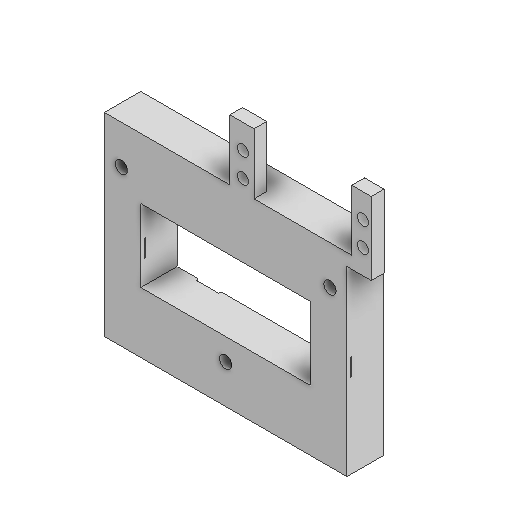
# Autodesk Inventor part: płytka_prowadzaca_rysik
Saved by Autodesk Inventor 2025.1 (Build 291241000, 241)
## iProperties
Created: 2025-04-08
Part Number: płytka_prowadzaca_rysik
Material: Ogólny
Document SubType Name: Modeling
Designer: Maciej
Density: 1 g/cm^3
Appearance: Domyślna
Author: Maciej
Autodesk Inventor part; units mm, degrees
ref_plane "YZ Plane" through (0, 0, 0) normal (1, 0, 0) x (0, 1, 0)
ref_plane "XZ Plane" through (0, 0, 0) normal (0, 1, 0) x (-1, 0, 0)
ref_plane "XY Plane" through (0, 0, 0) normal (0, 0, 1) x (1, 0, 0)
sketch "Szkic5" plane through (0, 0, 0) normal (0, 0, 1) x (1, 0, 0)
  line L0 (-50, -40) -> (50, -40)
  line L1 (50, -40) -> (50, 40)
  line L2 (50, 40) -> (-50, 40)
  line L3 (-50, 40) -> (-50, -40)
  line L4 (-50, -40) -> (50, 40) construction
  line L5 (50, -40) -> (-50, 40) construction
  line L6 (-35, -25) -> (35, -25)
  line L7 (35, -25) -> (35, 25)
  line L8 (35, 25) -> (-35, 25)
  line L9 (-35, 25) -> (-35, -25)
  line L10 (-35, -25) -> (35, 25) construction
  line L11 (35, -25) -> (-35, 25) construction
  point P0 (0, 0)
  dimension "d27" = 100
  dimension "d28" = 80
  dimension "d29" = 70
  dimension "d30" = 50
  constraints: 24 end point, 4 midpoint, 4 parallel, 2 horizontal, 2 perpendicular
  measures "d27" distance of L2.end L1.end
  measures "d28" distance of L1.end L0.end
  measures "d29" distance of L8.end L7.end
  measures "d30" distance of L7.end L6.end
extrude "Wyciągnięcie proste4" add sketch "Szkic5" against normal blind 13
sketch "Szkic6" plane through (0, 0, 0) normal (0, 0, 1) x (1, 0, 0)
  line L0 (-50, -40) -> (50, -40)
  line L1 (50, -40) -> (50, 40)
  line L2 (50, 40) -> (-50, 40)
  line L3 (-50, 40) -> (-50, -40)
  line L4 (-50, -40) -> (50, 40) construction
  line L5 (50, -40) -> (-50, 40) construction
  line L6 (35, -25) -> (35, 25) projected
  line L7 (-35, -25) -> (35, -25)
  line L8 (35, -25) -> (35, 25)
  line L9 (35, 25) -> (-35, 25)
  line L10 (-35, 25) -> (-35, -25)
  line L11 (-35, -25) -> (35, 25) construction
  line L12 (35, -25) -> (-35, 25) construction
  point P0 (0, 0)
  constraints: 24 end point, 4 midpoint, 4 parallel, 2 horizontal, 2 perpendicular
extrude "Wyciągnięcie proste5" add sketch "Szkic6" along normal blind 2
sketch "Szkic7" plane through (50, -40, -13) normal (1, 0, 0) x (0, 0, -1)
  line L0 (-13, 34.759) -> (-13.5, 34.759)
  line L1 (-13.5, 34.759) -> (-13.5, 41.759)
  line L2 (-13.5, 41.759) -> (-13, 41.759)
  line L3 (-13, 41.759) -> (-13, 34.759)
  line L4 (-13, 34.759) -> (-13.5, 41.759) construction
  line L5 (-13.5, 34.759) -> (-13, 41.759) construction
  line L6 (-15, 0) -> (-15, 80) projected
  line L7 (0, 80) -> (-15, 80) projected
  point P0 (-13, 40)
  point P1 (-13.25, 38.259)
  dimension "d35" = 0.5
  dimension "d36" = 7
  dimension "d37" = 1.5
  dimension "d38" = 41.741
  constraints: 12 end point, 2 midpoint, 2 parallel, 1 horizontal, 1 perpendicular
  measures "d35" distance of L1.end L2.end
  measures "d36" distance of L0.end L1.end
  measures "d37" distance between parallel lines of L6 L1
  measures "d38" distance from line of L7 point (-13.25, 38.259)
extrude "Wyciągnięcie proste6" cut sketch "Szkic7" against normal through all
sketch "Szkic8" plane through (-35, -25, -13) normal (0, 1, 0) x (1, 0, 0)
  line L0 (70, -15) -> (0, -15) projected
  line L1 (0, 0) -> (70, 0) projected
  line L2 (0, -15) -> (0, 0)
  line L3 (0, 0) -> (70, 0)
  line L4 (70, 0) -> (70, -15)
  line L5 (70, -15) -> (0, -15)
  point P0 (35, -13)
  constraints: 8 end point, 2 perpendicular, 1 collinear, 1 vertical
extrude "Wyciągnięcie proste7" add sketch "Szkic8" along normal blind 10
sketch "Szkic9" plane through (0, 0, 2) normal (0, 0, 1) x (1, 0, 0)
  line L0 (50, 40) -> (-50, 40) projected
  line L1 (-50, 40) -> (-50, -40) projected
  line L2 (50, -40) -> (50, 40) projected
  line L3 (-50, -40) -> (50, -40) projected
  point P0 (0, 0)
  point P1 (-43, 24)
  point P2 (43, 24)
  point P3 (0, -24.05)
  dimension "d43" = 16
  dimension "d44" = 16
  dimension "d45" = 7
  dimension "d46" = 7
  dimension "d54" = 15.95
  dimension "d55" = 50
  measures "d43" distance from line of L0 point (-43, 24)
  measures "d44" distance from line of L0 point (43, 24)
  measures "d45" distance from line of L1 point (-43, 24)
  measures "d46" distance from line of L2 point (43, 24)
  measures "d54" distance from line of L3 point (0, -24.05)
  measures "d55" distance from line of L1 point (0, -24.05)
hole "Otwór2" at (-43, 24, 2) at (43, 24, 2) at (0, -24.05, 2) direction (0, 0, -1) diameter 5 depth 15 clearance for "Śruba ze łbem płaskim obrobiona" size "M4" standard "ANSI Profil metryczny M"
sketch "Szkic10" plane through (0, 0, -13) normal (0, 0, -1) x (-1, 0, 0)
  line L0 (17, 31) -> (26, 31)
  line L1 (26, 31) -> (26, -39)
  line L2 (26, -39) -> (17, -39)
  line L3 (17, -39) -> (17, 31)
  line L4 (50, -40) -> (50, 40) projected
  line L5 (50, 40) -> (-50, 40) projected
  point P0 (0, 0)
  point P1 (21.5, 31)
  dimension "d56" = 9
  dimension "d57" = 70
  dimension "d58" = 24
  dimension "d59" = 9
  constraints: 8 end point, 2 parallel, 1 horizontal, 1 midpoint, 1 perpendicular
  measures "d56" distance of L1.end L2.end
  measures "d57" distance of L0.end L1.end
  measures "d58" distance between parallel lines of L4 L1
  measures "d59" distance from line of L5 point (21.5, 31)
extrude "Wyciągnięcie proste8" cut sketch "Szkic10" against normal blind 1
chamfer "Faza2" distance 0.5 angle 45 6 edges at (-21.5, -39, -13) (-17, -27, -13) (-26, -27, -13) (-17, 28, -13) (-21.5, 31, -13) (-26, 28, -13)
sketch "Szkic11" plane through (50, -40, -13) normal (1, 0, 0) x (0, 0, -1)
  line L0 (-15, 75) -> (-9.727, 75)
  line L1 (-9.727, 75) -> (-9.727, 105)
  line L2 (-9.727, 105) -> (-15, 105)
  line L3 (-15, 105) -> (-15, 75)
  line L4 (-15, 0) -> (-15, 80) projected
  line L5 (0, 80) -> (-15, 80) projected
  point P0 (-13, 40)
  point P1 (-7.5, 80)
  point P2 (-12.3635, 75)
  dimension "d68" = 5.273
  dimension "d69" = 30
  dimension "d71" = 5
  dimension "d74" = 5.273
  constraints: 8 end point, 2 midpoint, 2 parallel, 1 horizontal, 1 perpendicular
  measures "d68" distance of L2.end L1.end
  measures "d69" distance of L2.end L0.start
  measures "d71" vertical distance of point (-7.5, 80) point (-12.364, 75)
  measures "d74" distance between parallel lines of L4 L1
extrude "Wyciągnięcie proste9" add sketch "Szkic11" along normal blind 10
sketch "Szkic12" plane through (-50, 40, -13) normal (0, 1, 0) x (1, 0, 0)
  line L0 (61.698, -9.763) -> (51.698, -9.763)
  line L1 (51.698, -9.763) -> (51.698, -15)
  line L2 (51.698, -15) -> (61.698, -15)
  line L3 (61.698, -15) -> (61.698, -9.763)
  line L4 (100, 0) -> (100, -9.727) projected
  line L5 (100, -15) -> (0, -15) projected
  point P0 (50, -13)
  dimension "d75" = 10
  dimension "d76" = 5.237
  dimension "d77" = 38.302
  dimension "d78" = 0
  constraints: 8 end point, 2 parallel, 1 horizontal, 1 perpendicular
  measures "d75" distance of L2.end L1.end
  measures "d76" distance of L1.end L0.end
  measures "d77" distance between parallel lines of L4 L3
  measures "d78" distance between parallel lines of L5 L2
extrude "Wyciągnięcie proste10" add sketch "Szkic12" along normal up to surface (25 mm away)
sketch "Szkic14" plane through (50, -40, -13) normal (-1, 0, 0) x (0, 0, 1)
  line L0 (9.727, 105) -> (15, 105) projected
  line L1 (9.727, 105) -> (15, 105)
  line L2 (15, 105) -> (15, 80)
  line L3 (15, 80) -> (9.727, 80)
  line L4 (9.727, 80) -> (9.727, 105)
  point P0 (13, 40)
  constraints: 8 end point, 2 parallel, 1 horizontal, 1 perpendicular
extrude "Wyciągnięcie proste11" cut sketch "Szkic14" against normal blind 1.998
sketch "Szkic15" plane through (0, 0, 2) normal (0, 0, 1) x (1, 0, 0)
  line L0 (11.698, 65) -> (1.698, 65) projected
  line L1 (51.998, 65) -> (60, 65) projected
  line L2 (1.698, 40) -> (1.698, 65) projected
  line L3 (51.998, 65) -> (51.998, 40) projected
  line L4 (60, 65) -> (60, 35) projected
  point P0 (0, 0)
  point P1 (7.099, 55)
  point P2 (7.099, 45)
  point P3 (56.598, 55)
  point P4 (56.598, 45)
  point P5 (55.999, 65)
  point P6 (1.698, 52.5)
  dimension "d83" = 10
  dimension "d84" = 10
  dimension "d86" = 10
  dimension "d89" = 10
  dimension "d90" = 5.401
  dimension "d93" = 3.402
  dimension "d94" = 3.402
  constraints: 2 midpoint
  measures "d83" distance of point (7.099, 45) point (7.099, 55)
  measures "d84" distance of point (56.598, 45) point (56.598, 55)
  measures "d86" distance from line of L0 point (7.099, 55)
  measures "d89" distance from line of point (56.598, 55) L1
  measures "d90" horizontal distance of point (1.698, 52.5) point (7.099, 55)
  measures "d93" distance from line of L4 point (56.598, 55)
  measures "d94" distance from line of L4 point (56.598, 45)
hole "Otwór3" at (7.099, 55, 2) at (7.099, 45, 2) at (56.598, 55, 2) at (56.598, 45, 2) direction (0, 0, -1) diameter 4.5 depth 5.273 clearance for "Śruba ze łbem płaskim obrobiona" size "M4" standard "ANSI Profil metryczny M"
sketch "Szkic16" plane through (-35, 25, 2) normal (0, -1, 0) x (1, 0, 0)
  line L0 (70, -15) -> (18.5, -15) projected
  line L1 (70, -15) -> (0, -15)
  line L2 (0, -15) -> (0, 0)
  line L3 (0, 0) -> (70, 0)
  line L4 (70, 0) -> (70, -15)
  point P0 (35, -2)
  constraints: 8 end point, 2 parallel, 1 horizontal, 1 perpendicular
extrude "Wyciągnięcie proste12" add sketch "Szkic16" along normal blind 10
sketch "Szkic17" plane through (-35, 15, 2) normal (0, -1, 0) x (1, 0, 0)
  line L0 (8.5, -15) -> (18.5, -15) projected
  line L1 (18, -14) -> (18, -14.5) projected
  line L2 (18.5, -15) -> (18, -14.5)
  line L3 (18, -14.5) -> (18, -14)
  line L4 (9, -14) -> (18, -14) projected
  line L5 (18, -14) -> (9, -14)
  line L6 (9, -14) -> (9, -14.5)
  line L7 (9, -14.5) -> (8.5, -15)
  line L8 (8.5, -15) -> (18.5, -15)
  point P0 (35, -2)
  constraints: 12 end point, 3 perpendicular, 2 collinear
extrude "Wyciągnięcie proste13" cut sketch "Szkic17" against normal blind 10
equation "\"d44\" = d43"
equation "\"d46\" = d45"
equation "\"d68\" = d74"
equation "\"d94\" = d93"
